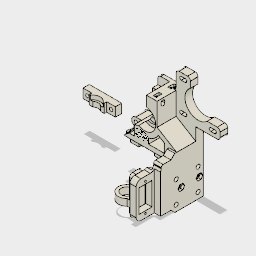
nixal_reprap4040_GregWadesReloaded (Autodesk Fusion 360 design; units mm, degrees)
Autodesk Fusion 360 part; units mm, degrees
sketch "nixal_bodyFront" plane through (0, 0, 0) normal (0, 0, 1) x (1, 0, 0)
  line L0 (33.2486, -0.8305) -> (33.2486, -67.8305)
  line L1 (25.2486, -26.17) -> (25.2486, -67.8305)
  line L2 (25.2486, -67.8305) -> (33.2486, -67.8305)
  circle A0 centre (35.6958, 20.1695) radius 13.75
  line L3 (12.6958, 37.912) -> (12.6958, 25.08)
  line L4 (33.2486, -13.9867) -> (12.6958, -1.5723)
  line L5 (20.378, -12.0924) -> (14.0147, -8.2249)
  arc A1 (3.655, -15.8336) -> (14.0147, -8.2249) centre (0, 0) ccw
  line L6 (3.655, -15.8336) -> (3.655, -21.42)
  line L7 (3.655, -21.42) -> (20.378, -21.42)
  line L8 (20.378, -21.42) -> (20.378, -12.0924)
  line L9 (-21.85, -26.17) -> (25.2486, -26.17)
  line L10 (12.15, -26.17) -> (12.15, -35.75)
  line L11 (12.15, -35.75) -> (-21.85, -35.75)
  circle A2 centre (0, 0) radius 11
  circle A3 centre (0, 0) radius 8
  arc A4 (-3.8595, -7.0074) -> (-1.9436, -3.6108) centre (-11.423, -0.5027) ccw
  arc A5 (-11.095, -10.9577) -> (-6.386, -9.2618) centre (-12.3813, 0) ccw
  line L12 (-4.45, -30.5) -> (-4.45, 30)
  line L13 (-11.095, -21.42) -> (-11.095, -2.5083)
  line L14 (-11.095, -10.9577) -> (-17.105, -10.9577)
  arc A6 (-17.105, -10.9577) -> (-19.716, -19.1129) centre (-17.105, -15.4532) ccw
  line L15 (-21.85, -25.42) -> (-16.4934, -21.42)
  line L16 (-16.4934, -21.42) -> (-19.716, -19.1129)
  line L17 (-11.095, -21.42) -> (-16.4934, -21.42)
  line L18 (-21.85, -35.75) -> (-21.85, -25.42)
  line L19 (-21.85, -28.75) -> (-26.35, -28.75)
  arc A7 (-26.35, -28.75) -> (-26.35, -35.75) centre (-26.35, -32.25) ccw
  circle A8 centre (-26.35, -32.25) radius 1.75
  line L20 (-11.095, 13.08) -> (1.4226, 13.08)
  line L21 (1.4226, 22.08) -> (1.4226, 3.8448)
  line L22 (12.6958, 22.08) -> (-8.095, 22.08)
  arc A9 (-8.095, 22.08) -> (-11.095, 19.08) centre (-8.095, 19.08) ccw
  line L23 (-11.095, 19.08) -> (-11.095, 2.5083)
  arc A10 (9.6958, 22.08) -> (12.6958, 25.08) centre (9.6958, 25.08) ccw
  arc A11 (15.6958, 40.912) -> (12.6958, 37.912) centre (15.6958, 37.912) ccw
  line L24 (15.6958, 40.912) -> (24.6958, 40.912)
  arc A12 (18.1458, 37.3695) -> (18.1458, 33.9695) centre (18.1458, 35.6695) ccw
  line L25 (18.1458, 33.9695) -> (22.2458, 33.9695)
  arc A13 (22.2458, 33.9695) -> (22.2458, 37.3695) centre (22.2458, 35.6695) ccw
  line L26 (22.2458, 37.3695) -> (18.1458, 37.3695)
  arc A14 (27.6958, 37.912) -> (24.6958, 40.912) centre (24.6958, 37.912) ccw
  line L27 (27.6958, 37.912) -> (27.6958, 31.3527)
  line L28 (12.6958, -1.5723) -> (12.6958, 22.08)
  line L29 (22.2458, 6.3695) -> (18.1458, 6.3695)
  arc A15 (18.1458, 6.3695) -> (18.1458, 2.9695) centre (18.1458, 4.6695) ccw
  line L30 (18.1458, 2.9695) -> (22.2458, 2.9695)
  arc A16 (22.2458, 2.9695) -> (22.2458, 6.3695) centre (22.2458, 4.6695) ccw
  line L31 (33.2486, -0.8305) -> (55.827, -0.8305)
  arc A17 (55.827, -0.8305) -> (58.827, 2.1695) centre (55.827, 2.1695) ccw
  line L32 (58.827, 7.1695) -> (58.827, 2.1695)
  arc A18 (58.827, 7.1695) -> (55.827, 10.1695) centre (55.827, 7.1695) ccw
  line L33 (45.1331, 10.1695) -> (55.827, 10.1695)
  line L34 (49.1458, 6.3695) -> (53.2458, 6.3695)
  arc A19 (53.2458, 2.9695) -> (53.2458, 6.3695) centre (53.2458, 4.6695) ccw
  circle A20 centre (7.65, -30.96) radius 1.75
  line L35 (7.65, -34.3375) -> (10.575, -32.6487)
  line L36 (4.725, -32.6487) -> (7.65, -34.3375)
  line L37 (4.725, -29.2713) -> (4.725, -32.6487)
  line L38 (7.65, -27.5825) -> (4.725, -29.2713)
  line L39 (10.575, -29.2713) -> (7.65, -27.5825)
  line L40 (10.575, -32.6487) -> (10.575, -29.2713)
  line L41 (-26.35, -35.75) -> (-21.85, -35.75)
  circle A21 centre (-17.35, -30.96) radius 1.75
  line L42 (-20.275, -29.2713) -> (-20.275, -32.6487)
  line L43 (-20.275, -32.6487) -> (-17.35, -34.3375)
  line L44 (-17.35, -34.3375) -> (-14.425, -32.6487)
  line L45 (-14.425, -32.6487) -> (-14.425, -29.2713)
  line L46 (-14.425, -29.2713) -> (-17.35, -27.5825)
  line L47 (-17.35, -27.5825) -> (-20.275, -29.2713)
  circle A22 centre (-17.105, -15.4532) radius 1.75
  line L48 (49.1458, 2.9695) -> (53.2458, 2.9695)
  arc A23 (49.1458, 6.3695) -> (49.1458, 2.9695) centre (49.1458, 4.6695) ccw
  arc A24 (-6.386, -9.2618) -> (-3.8595, -7.0074) centre (-12.3813, 0) ccw
  line L49 (-10.7102, -2.5083) -> (-11.095, -2.5083)
  line L50 (-11.095, 2.5083) -> (-10.7102, 2.5083)
  circle A25 centre (-0.0014, 0) radius 4.1
  line L51 (-11.095, 2.5083) -> (-11.095, -2.5083)
  dimension "d46" = 8.2
  dimension "d47" = 33.25
  dimension "d127" = 4.45
  constraint tangent L48 A23
  constraint coincident A25
  constraint coincident A1.centre A25
  constraint vertical L21
  constraint perpendicular L49 L51
  measures "d46" diameter of A25
  measures "d47" distance of L0 A1.centre
  measures "d127" distance of A1.centre L12
extrude "Extrude7" add sketch "nixal_bodyFront" along normal blind 27.5 contours L0 L1 L2 L4 L9 A2 L12 L21 L22 L28 | L9 A2 A5 L12 L13 L15 L17 L18 A24 makes body 1
extrude "Extrude8" add sketch "nixal_bodyFront" along normal blind 7.5 contours L0 A0 L3 L4 L22 A10 A11 L24 A14 L27 L28 L31 A17 L32 A18 L33 bodies 1
extrude "Extrude9" add sketch "nixal_bodyFront" along normal blind 3 contours L12 L20 L21 L22 | L12 L20 L22 A9 L23 bodies 1
extrude "Extrude10" add sketch "nixal_bodyFront" along normal blind 8.5 and the other way blind 0 contours A2 L12 L20 L21 | A2 A3 L12 L21 A24 | A2 L12 A24 | A2 L12 L20 L23 L50 | A2 A3 L12 L21 | A2 A5 L13 A24 L49 | A2 A3 L12 A24 | A3 L12 A24 | A3 A4 L12 L21 A25 | A3 A4 L21 A25 | A2 L49 L50 L51 | A3 L12 | A25 bodies 1
extrude "Extrude11" cut sketch "nixal_bodyFront" along normal blind 7.2 contours A2 A3 L12 L21 A24 | A2 L12 A24 | A2 A3 L12 L21 | A2 A3 L12 A24 | A3 L12 A24 | A3 A4 L12 L21 A25 | A3 A4 L21 A25 | A3 L12 | A25 bodies 1
extrude "Extrude12" add sketch "nixal_bodyFront" along normal blind 20.5 and the other way blind -8 separate body contours A2 A3 L12 L21 A24 | A2 L12 A24 makes body 2
sketch "Sketch5" plane through (0, -26.17, 0) normal (0, -1, 0) x (1, 0, 0)
  line L0 (-21.85, 0) -> (25.2486, 0)
  line L1 (25.2486, 0) -> (25.2486, 27.5)
  line L2 (25.2486, 27.5) -> (-21.85, 27.5)
  line L3 (-21.85, 27.5) -> (-21.85, 0)
  line L4 (-21.85, 13.75) -> (25.2486, 13.75) construction
  circle A0 centre (-4.0014, 13.75) radius 1.75
  line L5 (33.2486, 0) -> (33.2486, 27.5)
  circle A1 centre (-4.0014, 13.75) radius 6
  circle A2 centre (-4.0014, 13.75) radius 8
  line L6 (-12.0014, 13.75) -> (-12.0014, 27.5)
  line L7 (3.9986, 13.75) -> (3.9986, 27.5)
  line L8 (-10.0014, 13.75) -> (-10.0014, 27.5)
  line L9 (1.9986, 13.75) -> (1.9986, 27.5)
  line L10 (-12.0014, 27.5) -> (-10.0014, 27.5)
  line L11 (3.9986, 27.5) -> (1.9986, 27.5)
  line L12 (1.9986, 27.5) -> (-10.0014, 27.5)
  circle A3 centre (-4.0014, 13.75) radius 4.5
  dimension "d39" = 13.75
  dimension "d40" = 3.5
  dimension "d50" = 37.25
  dimension "d83" = 12
  dimension "d84" = 16
  dimension "d112" = 9
  constraint midpoint L3 origin
  constraint midpoint L1 origin
  constraint coincident L4 origin
  constraint concentric A0 A1
  constraint concentric A1 A2
  constraint coincident A2 origin
  constraint tangent A2 L6
  constraint tangent A2 L7
  constraint coincident L2 origin
  constraint coincident A1 origin
  constraint tangent A1 L8
  constraint tangent A1 L9
  constraint concentric A2 A3
  measures "d39" distance of L2 L4
  measures "d40" diameter of A0
  measures "d83" diameter of A1
  measures "d84" diameter of A2
  measures "d112" diameter of A3
extrude "Extrude15" add sketch "nixal_bodyFront" along normal blind 20 and the other way blind -8 contours L13 L14 A6 L16 L17 bodies 1
sketch "Sketch6" plane through (1.4226, 0, 0) normal (-1, 0, 0) x (0, 0, 1)
  line L0 (3, 13.08) -> (8.5, 13.08)
  line L1 (8.5, 13.08) -> (8.5, 10.9076)
  line L2 (8.5, 10.9076) -> (27.5, 10.9076)
  line L3 (27.5, 10.9076) -> (27.5, 22.08)
  line L4 (27.5, 22.08) -> (3, 22.08)
  line L5 (3, 22.08) -> (3, 13.08)
  line L6 (13.75, 24.9076) -> (13.75, 10.9076) construction
  line L7 (0, 19.08) -> (0, 2.5083)
  line L8 (4.5, 19.08) -> (4.5, 15.58)
  line L9 (8, 19.08) -> (8, 15.58)
  line L10 (19.5, 19.08) -> (19.5, 15)
  line L11 (23, 19.08) -> (23, 15)
  arc A0 (8, 19.08) -> (4.5, 19.08) centre (6.25, 19.08) ccw
  arc A1 (4.5, 15.58) -> (8, 15.58) centre (6.25, 15.58) ccw
  arc A2 (23, 19.08) -> (19.5, 19.08) centre (21.25, 19.08) ccw
  arc A3 (19.5, 15) -> (23, 15) centre (21.25, 15) ccw
  dimension "d54" = 13.75
  dimension "d55" = 14
  dimension "d56" = 3.5
  dimension "d57" = 3.5
  dimension "d58" = 7.5
  dimension "d59" = 7.5
  dimension "d60" = 3
  dimension "d61" = 3
  dimension "d62" = 3.5
  dimension "d63" = 7.5
  dimension "d64" = 3.5
  dimension "d65" = 3.5
  constraint perpendicular L4 L6
  constraint coincident L2 origin
  constraint tangent L8 A1
  constraint perpendicular L4 L8
  constraint tangent L9 A1
  constraint tangent L10 A3
  constraint vertical L10
  constraint tangent L11 A2
  constraint vertical L11
  measures "d54" distance of L3 L6
  measures "d55" distance of L6 L7
  measures "d56" diameter of A0
  measures "d57" diameter of A2
  measures "d58" distance of L6 origin
  measures "d59" distance of L6 origin
  measures "d62" diameter of A1
  measures "d63" distance of L6 origin
  measures "d65" diameter of A3
extrude "Extrude16" cut sketch "Sketch6" against normal blind 20 contours L10 L11 A2 A3 bodies 1
extrude "Extrude17" cut sketch "Sketch6" against normal blind 19 contours L8 L9 A0 A1 bodies 1
extrude "Extrude18" add sketch "nixal_bodyFront" along normal blind 19.5 and the other way blind -9 separate body contours A3 A4 L21 A25 makes body 3
extrude "Extrude19" cut sketch "nixal_bodyFront" along normal blind 19 contours A25 bodies 1
extrude "Extrude20" cut sketch "Sketch5" along normal blind -51 and the other way blind -25 contours A0 bodies 1 2 3
sketch "Sketch7" plane through (0, 22.08, 0) normal (0, 1, 0) x (-1, 0, 0)
  line L0 (-9.6958, 7.5) -> (-9.6958, 0)
  line L1 (-9.6958, 0) -> (8.095, 0)
  line L2 (8.095, 0) -> (8.095, 3)
  line L3 (8.095, 3) -> (-1.4226, 3)
  line L4 (-1.4226, 3) -> (-1.4226, 27.5)
  line L5 (-1.4226, 27.5) -> (-12.6958, 27.5)
  line L6 (-12.6958, 27.5) -> (-12.6958, 7.5)
  line L7 (-12.6958, 7.5) -> (-9.6958, 7.5)
  line L8 (-5, 3.1404) -> (-9, 3.1404)
  line L9 (-9, 3.1404) -> (-9, 9.1404)
  line L10 (-9, 9.1404) -> (-5, 9.1404)
  line L11 (-5, 9.1404) -> (-5, 3.1404)
  line L12 (-5, 17.8947) -> (-9, 17.8947)
  line L13 (-9, 17.8947) -> (-9, 23.8947)
  line L14 (-9, 23.8947) -> (-5, 23.8947)
  line L15 (-5, 23.8947) -> (-5, 17.8947)
  dimension "d76" = 6
  dimension "d77" = 6
  constraint horizontal L8
  constraint vertical L9
  constraint horizontal L10
  constraint vertical L11
  constraint horizontal L12
  constraint vertical L13
  constraint horizontal L14
  constraint vertical L15
  measures "d76" distance of L12 L14
  measures "d77" distance of L8 L10
extrude "Extrude21" cut sketch "Sketch7" against normal blind 11 contours L8 L9 L10 L11 | L12 L13 L14 L15 bodies 1
extrude "Extrude22" add sketch "nixal_bodyFront" along normal blind 21 contours L9 L10 L11 L18 | L35 L36 L37 L38 L39 L40 | L42 L43 L44 L45 L46 L47 bodies 1
extrude "Extrude23" cut sketch "Sketch5" along normal blind 4 contours L2 A2 L6 L8 L10 | L2 A2 L7 L9 L11 | A1 A2 L8 L9 picked at (3.2798, 13.0545) bodies 1
extrude "Extrude24" cut sketch "Sketch5" along normal blind 13 and the other way blind 0 contours L2 A2 L8 L9 L12 | A1 A2 L8 L9 | A1 | A0 | A3 picked at (-4.5265, 21.0511) bodies 1
extrude "Extrude25" add sketch "nixal_bodyFront" along normal blind 17.75 and the other way blind -9.75 contours L18 L19 A7 L41 bodies 1
sketch "Sketch8" plane through (33.2486, 0, 0) normal (1, 0, 0) x (0, 0, -1)
  line L0 (0, -67.8305) -> (0, -0.8305)
  line L1 (0, -0.8305) -> (-7.5, -0.8305)
  line L2 (-7.5, -0.8305) -> (-7.5, -13.9867)
  line L3 (-7.5, -13.9867) -> (-27.5, -13.9867)
  line L4 (-27.5, -13.9867) -> (-27.5, -67.8305)
  line L5 (-27.5, -67.8305) -> (0, -67.8305)
  line L6 (-28, -18) -> (-5, -18)
  line L7 (-5, -18) -> (-5, -41)
  line L8 (-5, -41) -> (-28, -41)
  line L9 (-28, -41) -> (-28, -18)
  line L10 (0, -26) -> (-27.5, -26)
  line L11 (-27.5, -13.9867) -> (-33.5, -13.9867)
  line L12 (-33.5, -13.9867) -> (-33.5, -47.9867)
  line L13 (-33.5, -47.9867) -> (-27.5, -47.9867)
  line L14 (-27.5, -47.9867) -> (-27.5, -13.9867)
  circle A0 centre (-5, -18) radius 2.15
  circle A1 centre (-28, -18) radius 2.15
  circle A2 centre (-28, -41) radius 2.15
  circle A3 centre (-5, -41) radius 2.15
  circle A4 centre (-28, -32) radius 2.15
  circle A5 centre (-5, -32) radius 2.15
  line L15 (-27.5, -47.9867) -> (0, -47.9867)
  dimension "d95" = 23
  dimension "d96" = 23
  dimension "d97" = 5
  dimension "d98" = 8
  dimension "d99" = 6
  dimension "d100" = 34
  dimension "d101" = 4.3
  dimension "d102" = 4.3
  dimension "d103" = 4.3
  dimension "d104" = 4.3
  dimension "d109" = 4.3
  dimension "d110" = 9
  dimension "d111" = 4.3
  constraint horizontal L6
  constraint vertical L7
  constraint horizontal L8
  constraint vertical L9
  constraint coincident L0 origin
  constraint coincident L4 origin
  constraint perpendicular L4 L10
  constraint horizontal L11
  constraint vertical L12
  constraint horizontal L13
  constraint vertical L14
  constraint coincident L9
  constraint coincident L7
  constraint coincident L0
  constraint perpendicular L0 L15
  measures "d97" distance of L0 L7
  measures "d100" distance of origin
  measures "d101" diameter of A0
  measures "d102" diameter of A1
  measures "d103" diameter of A2
  measures "d104" diameter of A3
  measures "d109" diameter of A4
  measures "d110" distance of origin
  measures "d111" diameter of A5
extrude "Extrude26" add sketch "Sketch8" against normal blind 8 contours L4 L9 L11 L12 L13 L14 A1 A2 A4 | L4 L8 L9 L14 A2 | L4 L9 L14 A1 A4 | L4 L8 L9 L14 A2 | L4 L9 L14 A2 A4 | L4 L6 L9 L14 A1 | L4 L9 L14 A4 | L9 A4 | L4 L6 L9 L14 A1 bodies 1
extrude "Extrude27" cut sketch "Sketch8" against normal blind 16 contours L4 L8 L9 L14 A2 | L4 L8 L14 A2 | L6 L7 A0 | L6 L7 A0 | L7 A5 | L7 A5 | L4 L8 L9 L14 A2 | L4 L8 L14 A2 | L4 L6 L9 L14 A1 | L4 L6 L14 A1 | L4 L14 A4 | L4 L9 L14 A4 | L9 A4 | L7 L8 A3 | L7 L8 A3 | L4 L6 L14 A1 | L4 L6 L9 L14 A1 bodies 1
extrude "Extrude28" cut sketch "Sketch5" against normal blind 5 contours A3 bodies 1
sketch "Sketch9" plane through (0, 0, 33.5) normal (0, 0, 1) x (1, 0, 0)
  line L0 (33.2486, -47.9867) -> (33.2486, -13.9867)
  line L1 (33.2486, -13.9867) -> (25.2486, -13.9867)
  line L2 (25.2486, -13.9867) -> (25.2486, -47.9867)
  line L3 (25.2486, -47.9867) -> (33.2486, -47.9867)
  line L4 (27.1542, -14.3315) -> (31.1542, -14.3315)
  line L5 (31.1542, -14.3315) -> (31.1542, -21.8315)
  line L6 (31.1542, -21.8315) -> (27.1542, -21.8315)
  line L7 (27.1542, -21.8315) -> (27.1542, -14.3315)
  dimension "d115" = 4
  dimension "d116" = 7.5
  constraint horizontal L4
  constraint vertical L5
  constraint horizontal L6
  constraint vertical L7
extrude "Extrude29" cut sketch "Sketch9" against normal blind 11 contours L4 L5 L6 L7 bodies 1
extrude "Extrude30" cut sketch "Sketch9" along normal blind -34 and the other way blind 24 contours L4 L5 L6 L7 bodies 1
move_face "OffsetFaces1" offset 2 1 faces at (30.582, -13.9867, 29.5) on bodies 1
extrude "Extrude31" cut 1 faces at (32.1449, -12.6533, 27.5) along direction (0, 0, 1) blind 10 on bodies 1 bodies 1
extrude "Extrude32" cut sketch "Sketch8" against normal blind 39 contours L0 L4 L5 L15 bodies 1
equation "centersFilament2hobbed = 4 mm"
equation "backwall = 8 mm"
equation "hobbed2wall = 33.25 mm"
equation "d50 = hobbed2wall + centersFilament2hobbed"
